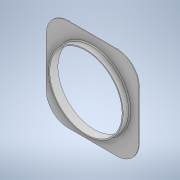
# Autodesk Inventor part: SolarGearBearing
Saved by Autodesk Inventor 2021 (Build 250183000, 183)
## iProperties
Created: 2021-02-06
Part Number: SolarGearBearing
Material: Generic
Document SubType Name: Sheet Metal
Designer: allen
Density: 1 g/cm^3
Sheet Metal Rule: Default_mm
Appearance: Default
Author: allen
Autodesk Inventor part; units mm, degrees
ref_plane "YZ Plane" through (0, 0, 0) normal (1, 0, 0) x (0, 1, 0)
ref_plane "XZ Plane" through (0, 0, 0) normal (0, 1, 0) x (-1, 0, 0)
ref_plane "XY Plane" through (0, 0, 0) normal (0, 0, 1) x (1, 0, 0)
sketch "Sketch2" plane through (0, 0, 0) normal (0, 0, 1) x (1, 0, 0)
  line L0 (85, -85) -> (-85, -85)
  line L1 (-85, -85) -> (-85, 85)
  line L2 (-85, 85) -> (85, 85)
  line L3 (85, 85) -> (85, -85)
  line L4 (85, -85) -> (-85, 85) construction
  line L5 (-85, -85) -> (85, 85) construction
  circle A0 centre (0, 0) radius 68.5
  dimension "d3" = 170
  dimension "d4" = 170
  dimension "d5" = 137
  constraints: 12 end point, 2 midpoint, 2 parallel, 1 centre point, 1 coincident, 1 horizontal, 1 perpendicular
  measures "d3" distance of L1.end L2.end
  measures "d4" distance of L0.end L1.end
  measures "d5" diameter of A0
extrude "Extrusion1" add sketch "Sketch2" along normal blind 3
fillet "Fillet1" radius 40 4 edges at (85, 85, 1.5) (85, -85, 1.5) (-85, -85, 1.5) (-85, 85, 1.5)
sketch "Sketch3" plane through (0, 0, 0) normal (0, 0, 1) x (1, 0, 0)
  circle A0 centre (0, 0) radius 66.5
  circle A1 centre (0, 0) radius 68.5
  circle A2 centre (0, 0) radius 68.5
  dimension "d9" = 133
  dimension "d10" = 137
  constraints: 3 centre point, 3 coincident, 1 concentric
  measures "d9" diameter of A0
  measures "d10" diameter of A1
extrude "Extrusion2" add sketch "Sketch3" along normal blind 15
fillet "Fillet3" radius 2 1 edges at (-68.5, 0, 3)
fillet "Fillet4" radius 2 8 edges at (85, 0, 0) (73.2843, 73.2843, 0) (0, 85, 0) (-73.2843, 73.2843, 0) (-85, 0, 0) (-73.2843, -73.2843, 0) (0, -85, 0) (73.2843, -73.2843, 0)
equation "\"BendRadius\" = Thickness"
equation "\"BendReliefWidth\" = Thickness"
equation "\"BendReliefDepth\" = 0.5 * Thickness"
equation "\"CornerReliefSize\" = 4 * Thickness"
equation "\"MinimumRemnant\" = 2 * Thickness"
equation "\"TransitionRadius\" = BendRadius"
equation "\"JacobiRadiusSize\" = BendRadius"
equation "\"GapSize\" = Thickness"
equation "\"Thickness\" = 0.5"
body "Solid1"
